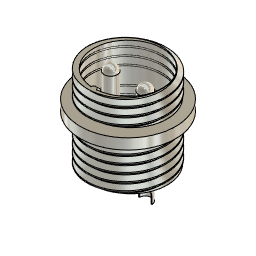
StarTopper (Autodesk Fusion 360 archive; units mm, degrees)
design "PowerConnector"
Autodesk Fusion 360 part; units mm, degrees
sketch "Sketch1" plane through (0, 0, 0) normal (0, 0, 1) x (1, 0, 0) in component "PowerConnector"
  circle A0 centre (0, 0) radius 7.5
  circle A1 centre (0, 0) radius 6.5
  arc A2 (0.997, -6.4231) -> (-0.997, -6.4231) centre (0, -6.5) ccw
  line L0 (-7.5, 0) -> (-3.25, 0) construction
  line L1 (7.5, 0) -> (3.25, 0) construction
  circle A3 centre (-3.25, 0) radius 1.25
  circle A4 centre (3.25, 0) radius 1.25
  circle A5 centre (0, 0) radius 9
  dimension "d1" = 15
  dimension "d2" = 13
  dimension "d3" = 2
  dimension "d5" = 4.25
  dimension "d6" = 4.25
  dimension "d7" = 2.5
  dimension "d8" = 2.5
  dimension "d9" = 18
  constraint coincident A0.centre A1.centre
  constraint coincident A1 A2.centre
  constraint coincident A1 A2.start
  constraint coincident A1 A2.end
  constraint coincident A0 L0.start
  constraint horizontal L0
  constraint coincident A0 L1.start
  constraint horizontal L1
  constraint coincident L0.end A3.centre
  constraint coincident L1.end A4.centre
  constraint concentric A1 A5
  measures "d1" diameter of A0
  measures "d2" diameter of A1
  measures "d3" diameter of A2
  measures "d5" distance of L0.start L0.end
  measures "d6" distance of L1.start L1.end
  measures "d7" diameter of A3
  measures "d8" diameter of A4
  measures "d9" diameter of A5
extrude "Extrude1" add sketch "Sketch1" along normal blind 5 contours A0 | A1 A2 picked at (0, -6.161) makes body 1 in component "PowerConnector"
extrude "Extrude2" add sketch "Sketch1" against normal blind 2 separate body contours A5 makes body 2 in component "PowerConnector"
extrude "Extrude3" add sketch "Sketch1" along normal blind 4.2 separate body contours A3 | A4 makes body 3 at (-2.0062, -0.1245, 1.4) makes body 4 at (4.4938, -0.1245, 1.4) in component "PowerConnector"
fillet "Fillet1" radius 1.25 2 edges at (-4.4154, -0.452, 4.2) (2.0846, -0.452, 4.2) on bodies 3 4 in component "PowerConnector"
chamfer "Chamfer1" distance 0.5 angle 45 1 edges at (0, -5.5, 5) on bodies 1 in component "PowerConnector"
extrude "Extrude4" add sketch "Sketch1" against normal blind 10.8 contours A0 bodies 1 2 in component "PowerConnector"
extrude "Extrude5" add sketch "Sketch1" against normal blind 9.8 separate body contours A1 A2 picked at (-0.1011, 2.7311) makes body 5 in component "PowerConnector"
extrude "Extrude6" add sketch "Sketch1" against normal blind 15 contours A3 | A4 bodies 3 4 5 in component "PowerConnector"
extrude "Extrude7" add sketch "Sketch1" against normal blind 9.8 contours A1 A2 picked at (0, -6.161) bodies 1 3 in component "PowerConnector"
sketch "Sketch2" plane through (0, 0, -15) normal (0, 0, -1) x (1, 0, 0) in component "PowerConnector"
  circle A0 centre (-3.25, 0) radius 1.25
  circle A1 centre (-3.25, 0) radius 1.1
  circle A2 centre (3.25, 0) radius 1.1
  circle A3 centre (3.25, 0) radius 1.25
  dimension "d27" = 2.2
  dimension "d28" = 2.2
  constraint concentric A0 A1
  constraint concentric A2 A3
  measures "d27" diameter of A1
  measures "d28" diameter of A2
extrude "Extrude8" cut sketch "Sketch2" against normal blind 3 contours A1 | A2 bodies 1 in component "PowerConnector"
sketch "Sketch3" plane through (0, 0, -15) normal (0, 0, -1) x (1, 0, 0) in component "PowerConnector"
  circle A0 centre (-3.25, 0) radius 1.1
  circle A1 centre (-3.25, 0) radius 1.25
  line L0 (-4.5, 0) -> (-2, 0)
  constraint coincident A1 L0.start
  constraint coincident A1 L0.end
  constraint horizontal L0
extrude "Extrude9" cut sketch "Sketch3" against normal blind 2.5 contours A0 A1 L0 picked at (-4.2726, 0.6221) bodies 1 in component "PowerConnector"
sketch "Sketch4" plane through (0, 0, -15) normal (0, 0, -1) x (1, 0, 0) in component "PowerConnector"
  circle A0 centre (3.25, 0) radius 1.1
  circle A1 centre (3.25, 0) radius 1.25
  line L0 (2, 0) -> (4.5, 0)
  constraint coincident A1 L0.start
  constraint coincident A1 L0.end
  constraint horizontal L0
extrude "Extrude10" cut sketch "Sketch4" against normal blind 2.5 contours A0 A1 L0 picked at (4.4413, 0.1167) bodies 1 in component "PowerConnector"
fillet "Fillet2" radius 1.1 4 edges at (-4.425, 0, -12.5) (-2.075, 0, -12.5) (2.075, 0, -12.5) (4.425, 0, -12.5) on bodies 1 in component "PowerConnector"
thread "Thread1" "ISO Metric profile 15.0 M15x1.5 6g" major diameter 14.85 minor diameter 13.1369 pitch 1.5 angle 60 modelled right hand crest width 0.2152 on face at (7.4907, -0.3738, 3.3333) crest through (7.425, 0, -0.375) on face at (7.4627, -0.7468, -4.9333) crest through (7.425, 0, -11.175) on bodies 1 in component "PowerConnector"
extrude "Extrude11" cut 1 faces at (0, 2.7335, 0) along direction (0, 0, -1) blind 5.2 on bodies 1 bodies 1 in component "PowerConnector"
component "PowerConnector" placed x (1, 0, 0) y (0, 1, 0) z (0, 0, 1) at (0, 0, 0)
equation "d23 = -9.80 mm - 5.2 mm"
